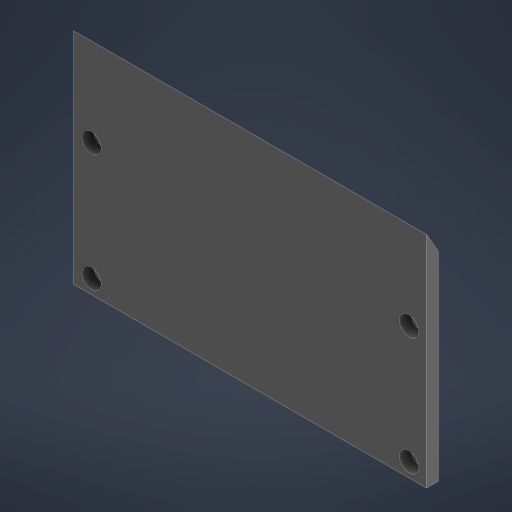
# Autodesk Inventor part: obciążenie_dół
Saved by Autodesk Inventor 2023.4 (Build 274418000, 418)
## iProperties
Created: 2025-10-31
Part Number: obciążenie_dół
Material: Stal
Document SubType Name: Modeling
Designer: Jakub Borsukiewicz
Density: 7.85 g/cm^3
Appearance: Szara
Author: Jakub Borsukiewicz
Autodesk Inventor part; units mm, degrees
ref_plane "YZ Plane" through (0, 0, 0) normal (1, 0, 0) x (0, 1, 0)
ref_plane "XZ Plane" through (0, 0, 0) normal (0, 1, 0) x (-1, 0, 0)
ref_plane "XY Plane" through (0, 0, 0) normal (0, 0, 1) x (1, 0, 0)
sketch "Szkic1" plane through (0, 0, 0) normal (0, 0, 1) x (1, 0, 0)
  line L0 (0, -39.2) -> (0, 39.2) projected
  line L1 (-63, 0) -> (63, 0) projected
  line L2 (-45, -28) -> (45, -28)
  line L3 (45, -28) -> (45, 28)
  line L4 (45, 28) -> (-45, 28)
  line L5 (-45, 28) -> (-45, -28)
  line L6 (-45, -28) -> (45, 28) construction
  line L7 (45, -28) -> (-45, 28) construction
  point P0 (0, 0)
  dimension "d0" = 90
  dimension "d1" = 56
  constraints: 12 end point, 2 midpoint, 2 parallel, 1 horizontal, 1 perpendicular
  measures "d0" distance of L3.end L4.end
  measures "d1" distance of L2.end L3.end
extrude "Wyciągnięcie proste1" add sketch "Szkic1" along normal blind 3
sketch "Szkic2" plane through (45, -28, 0) normal (1, 0, 0) x (0, 0, -1)
  line L0 (-3, 0) -> (-3, 56) projected
  line L1 (-3, 56) -> (0, 50.8038)
  line L2 (0, 0) -> (0, 56) projected
  line L3 (0, 0) -> (0, 56) projected
  line L4 (0, 56) -> (-3, 56) projected
  line L5 (-3, 0) -> (-3, 56) projected
  line L6 (0, 0) -> (-3, 0) projected
  point P0 (0, 28)
  dimension "d4" = 30
  constraints: 2 end point, 1 point on line
  measures "d4" angle of L0 L1
extrude "Wyciągnięcie proste2" cut sketch "Szkic2" against normal blind 90 contours L4 L2 L1
sketch "Szkic3" plane through (0, 0, 3) normal (0, 0, 1) x (1, 0, 0)
  line L0 (-45, -28) -> (45, -28) projected
  line L1 (45, -28) -> (45, 28) projected
  line L2 (45, 28) -> (-45, 28) projected
  line L3 (-45, 28) -> (-45, -28) projected
  point P0 (0, 0)
  point P1 (40.5, 5.5)
  point P2 (40.5, -24.5)
  dimension "d7" = 4.5
  dimension "d8" = 4.5
  dimension "d9" = 3.5
  dimension "d10" = 30
  measures "d7" distance from line of L1 point (40.5, -24.5)
  measures "d8" distance from line of L1 point (40.5, 5.5)
  measures "d9" distance from line of L0 point (40.5, -24.5)
  measures "d10" distance of point (40.5, -24.5) point (40.5, 5.5)
hole "Otwór1" at (40.5, 5.5, 3) at (40.5, -24.5, 3) direction (0, 0, -1) diameter 5 depth 3
mirror "Odbij1" about plane through (0, 0, 0) normal (1, 0, 0) of "Otwór1"
